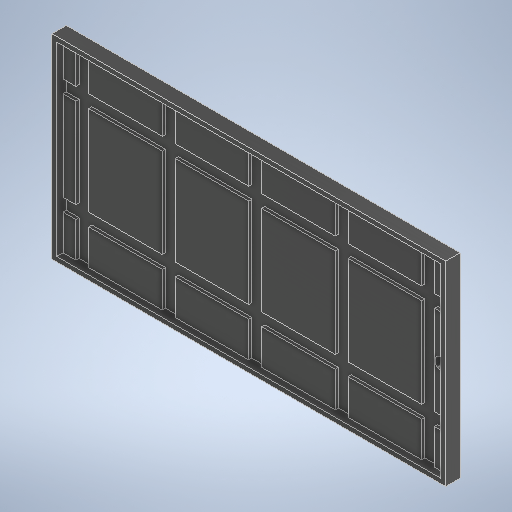
# Autodesk Inventor part: flood tray
Saved by Autodesk Inventor 2025 (Build 290162000, 162)
## iProperties
Created: 2024-06-19
Part Number: flood tray
Material: Generic
Document SubType Name: Modeling
Designer: Isaac
Density: 1 g/cm^3
Appearance: Dark Gray
Author: Isaac
Autodesk Inventor part; units mm, degrees
ref_plane "YZ Plane" through (0, 0, 0) normal (1, 0, 0) x (0, 1, 0)
ref_plane "XZ Plane" through (0, 0, 0) normal (0, 1, 0) x (-1, 0, 0)
ref_plane "XY Plane" through (0, 0, 0) normal (0, 0, 1) x (1, 0, 0)
sketch "Sketch1" plane through (0, 0, 0) normal (0, 0, 1) x (1, 0, 0)
  line L0 (-615, 305) -> (615, 305)
  line L1 (615, 305) -> (615, -305)
  line L2 (615, -305) -> (-615, -305)
  line L3 (-615, -305) -> (-615, 305)
  line L4 (-615, 305) -> (615, -305) construction
  line L5 (615, 305) -> (-615, -305) construction
  point P0 (0, 0)
  dimension "d0" = 610
  dimension "d1" = 1230
  constraints: 12 end point, 2 midpoint, 2 parallel, 1 horizontal, 1 perpendicular
  measures "d0" distance of L2.end L0.start
  measures "d1" distance of L0.start L0.end
extrude "Extrusion1" add sketch "Sketch1" along normal blind 45
sketch "Sketch2" plane through (0, 0, 45) normal (0, 0, 1) x (1, 0, 0)
  line L0 (-600, 290) -> (600, 290)
  line L1 (600, 290) -> (600, -290)
  line L2 (600, -290) -> (-600, -290)
  line L3 (-600, -290) -> (-600, 290)
  line L4 (-600, 290) -> (600, -290) construction
  line L5 (600, 290) -> (-600, -290) construction
  point P0 (0, 0)
  dimension "d4" = 1200
  dimension "d5" = 580
  constraints: 12 end point, 2 midpoint, 2 parallel, 1 horizontal, 1 perpendicular
  measures "d4" distance of L0.start L0.end
  measures "d5" distance of L0.end L1.end
extrude "Extrusion2" cut sketch "Sketch2" against normal blind 20
sketch "Sketch3" plane through (0, 0, 25) normal (0, 0, 1) x (1, 0, 0)
  line L0 (-20, 290) -> (20, 290)
  line L1 (20, 290) -> (20, -290)
  line L2 (20, -290) -> (-20, -290)
  line L3 (-20, -290) -> (-20, 290)
  line L4 (-20, 290) -> (20, -290) construction
  line L5 (20, 290) -> (-20, -290) construction
  line L6 (250, 290) -> (290, 290)
  line L7 (290, 290) -> (290, -290)
  line L8 (290, -290) -> (250, -290)
  line L9 (250, -290) -> (250, 290)
  line L10 (-290, 290) -> (-250, 290)
  line L11 (-250, 290) -> (-250, -290)
  line L12 (-250, -290) -> (-290, -290)
  line L13 (-290, -290) -> (-290, 290)
  line L14 (-600, 290) -> (600, 290) projected
  line L15 (520, 290) -> (560, 290)
  line L16 (560, 290) -> (560, -290)
  line L17 (560, -290) -> (520, -290)
  line L18 (520, -290) -> (520, 290)
  line L19 (-560, 290) -> (-520, 290)
  line L20 (-520, 290) -> (-520, -290)
  line L21 (-520, -290) -> (-560, -290)
  line L22 (-560, -290) -> (-560, 290)
  point P0 (0, 0)
  point P1 (250, 0)
  point P2 (-250, 0)
  point P3 (520, 0)
  point P4 (290, 0)
  point P5 (-290, 0)
  point P6 (-520, 0)
  dimension "d8" = 580
  dimension "d9" = 40
  dimension "d10" = 250
  dimension "d11" = 40
  dimension "d12" = 40
  dimension "d13" = 250
  dimension "d14" = 40
  dimension "d15" = 230
  dimension "d16" = 580
  dimension "d17" = 40
  dimension "d18" = 230
  constraints: 44 end point, 10 parallel, 8 midpoint, 5 horizontal, 5 perpendicular, 2 other
  measures "d8" distance of L0.end L1.end
  measures "d9" distance of L0.start L0.end
  measures "d10" distance of point (250, 0) point (0, 0)
  measures "d11" distance between parallel lines of L7 L9
  measures "d12" distance of L10.start L10.end
  measures "d13" distance of point (0, 0) point (-250, 0)
  measures "d14" distance of L16.end L17.end
  measures "d15" distance of point (520, 0) point (290, 0)
  measures "d16" distance of L21.end L19.start
  measures "d17" distance of L20.end L21.end
  measures "d18" distance of point (-290, 0) point (-520, 0)
extrude "Extrusion3" cut sketch "Sketch3" against normal blind 10
sketch "Sketch4" plane through (0, 0, 25) normal (0, 0, 1) x (1, 0, 0)
  line L0 (600, 290) -> (600, -290) projected
  line L1 (-600, 180) -> (600, 180)
  line L2 (600, 180) -> (600, 140)
  line L3 (600, 140) -> (-600, 140)
  line L4 (-600, 140) -> (-600, 180)
  line L5 (-600, -140) -> (600, -140)
  line L6 (600, -140) -> (600, -180)
  line L7 (600, -180) -> (-600, -180)
  line L8 (-600, -180) -> (-600, -140)
  point P0 (0, 0)
  point P1 (0, 140)
  point P2 (0, -140)
  point P3 (600, -140)
  dimension "d21" = 140
  dimension "d22" = 140
  dimension "d23" = 40
  dimension "d24" = 40
  dimension "d25" = 1200
  constraints: 16 end point, 4 parallel, 3 point on line, 2 horizontal, 2 midpoint, 2 perpendicular
  measures "d21" distance of point (0, 140) point (0, 0)
  measures "d22" distance of point (0, -140) point (0, 0)
  measures "d23" distance between parallel lines of L3 L1
  measures "d24" distance between parallel lines of L7 L5
  measures "d25" distance of L1.start L1.end
extrude "Extrusion4" cut sketch "Sketch4" against normal blind 10
sketch "Sketch5" plane through (0, 0, 25) normal (0, 0, 1) x (1, 0, 0)
  circle A0 centre (580, 0) radius 18.5
  point P0 (0, 0)
  dimension "d28" = 37
  dimension "d29" = 580
  constraints: 1 centre point
  measures "d28" diameter of A0
  measures "d29" distance of point (0, 0) A0.centre
extrude "Extrusion5" cut sketch "Sketch5" against normal blind 37
equation "\"d30\" = d28"
body "Solid1"
